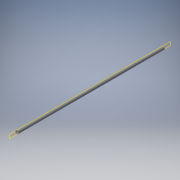
# Autodesk Inventor part: roundCatapultArm
Saved by Autodesk Inventor 2016 SP1 (Build 200210100, 210)
## iProperties
Created: 2016-01-18
Part Number: roundCatapultArm
Material: Generic
Document SubType Name: Modeling
Designer: steele
Density: 1 g/cm^3
Appearance: Default
Author: steele
Autodesk Inventor part; units mm, degrees
ref_plane "XY Plane" through (0, 0, 0) normal (0, 0, 1) x (1, 0, 0)
sketch "Sketch1" plane through (0, 0, 0) normal (0, 0, 1) x (1, 0, 0)
  circle A0 centre (0, 0) radius 11.43
  circle A1 centre (0, 0) radius 13.97
  dimension "d0" = 27.94
  dimension "d1" = 22.86
  constraints: 2 centre point, 2 coincident
  measures "d0" diameter of A1
  measures "d1" diameter of A0
extrude "Extrusion1" add sketch "Sketch1" along normal blind 1219.2
ref_plane "Work Plane3" through (13.97, 0, 0) normal (1, 0, 0) x (0, 1, 0)
sketch "Sketch3" plane through (13.97, 0, 0) normal (1, 0, 0) x (0, 1, 0)
  circle A0 centre (0, 1092.2) radius 3.175
  line L0 (13.97, 1219.2) -> (-13.97, 1219.2) projected
  point P0 (0, 0)
  dimension "d5" = 127
  dimension "d6" = 6.35
  constraints: 1 centre point
  measures "d5" distance from line of A0.centre L0
  measures "d6" diameter of A0
extrude "Extrusion2" cut sketch "Sketch3" against normal through all
ref_plane "Work Plane4" through (0, 13.97, 0) normal (0, 1, 0) x (-1, 0, 0)
sketch "Sketch4" plane through (0, 13.97, 0) normal (0, 1, 0) x (-1, 0, 0)
  circle A0 centre (0, 1193.8) radius 3.175
  line L0 (13.97, 1219.2) -> (-13.97, 1219.2) projected
  point P0 (0, 0)
  dimension "d9" = 6.35
  dimension "d10" = 25.4
  constraints: 1 centre point
  measures "d9" diameter of A0
  measures "d10" distance from line of A0.centre L0
extrude "Extrusion3" cut sketch "Sketch4" against normal through all
equation "\"d1\" = cArmInsideDiam"
equation "\"d5\" = cArmAxelDistanceFromEnd"
equation "\"d6\" = boltHolesDiam"
equation "\"d9\" = boltHolesDiam"
equation "\"d10\" = cArmHingeDistanceFromEnd"
equation "\"cArmAxelDistanceFromEnd\" = 127"
equation "\"cArmOutsideDiam\" = 27.94"
equation "\"cArmInsideDiam\" = 22.86"
equation "\"cArmLength\" = 1219.2"
equation "\"boltHolesDiam\" = 6.35"
equation "\"cArmHingeDistanceFromEnd\" = 25.4"
body "Solid1"
